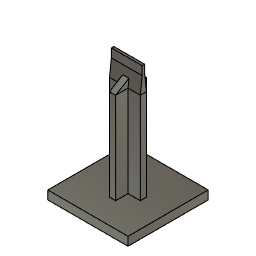
Base apoio braço (Autodesk Fusion 360 design; units mm, degrees)
Autodesk Fusion 360 part; units mm, degrees
sketch "Sketch1" plane through (0, 0, 0) normal (0, 0, 1) x (1, 0, 0)
  line L0 (0, 0) -> (65, 0)
  line L1 (65, 0) -> (65, 65)
  line L2 (65, 65) -> (0, 65)
  line L3 (0, 65) -> (0, 0)
  line L4 (20, 30) -> (45, 30)
  line L5 (45, 30) -> (45, 35)
  line L6 (45, 35) -> (20, 35)
  line L7 (20, 35) -> (20, 30)
  line L8 (30, 20) -> (35, 20)
  line L9 (35, 20) -> (35, 45)
  line L10 (35, 45) -> (30, 45)
  line L11 (30, 45) -> (30, 20)
  dimension "d1" = 65
  dimension "d2" = 65
  dimension "d3" = 25
  dimension "d4" = 5
  dimension "d5" = 5
  dimension "d6" = 25
  constraint horizontal L0
  constraint vertical L1
  constraint horizontal L2
  constraint vertical L3
  constraint coincident L0.start L3.end
  constraint horizontal L4
  constraint vertical L5
  constraint horizontal L6
  constraint vertical L7
  constraint horizontal L8
  constraint vertical L9
  constraint horizontal L10
  constraint vertical L11
  measures "d1" distance of L0.start L0.end
  measures "d2" distance of L0.start L2.end
  measures "d3" distance of L4.start L4.end
  measures "d4" distance of L4.start L6.end
  measures "d5" distance of L8.start L8.end
  measures "d6" distance of L8.start L10.end
extrude "Extrude1" add sketch "Sketch1" against normal blind 7 makes body 1
sketch "Sketch2" plane through (0, 0, 0) normal (0, 0, 1) x (-1, 0, 0)
  line L0 (-30, -35) -> (-30, -45)
  line L1 (-30, -45) -> (-35, -45)
  line L2 (-35, -45) -> (-35, -35)
  line L3 (-35, -35) -> (-45, -35)
  line L4 (-45, -35) -> (-45, -30)
  line L5 (-45, -30) -> (-35, -30)
  line L6 (-35, -30) -> (-35, -20)
  line L7 (-35, -20) -> (-30, -20)
  line L8 (-30, -20) -> (-30, -30)
  line L9 (-30, -30) -> (-20, -30)
  line L10 (-20, -30) -> (-20, -35)
  line L11 (-20, -35) -> (-30, -35)
  line L12 (0, -65) -> (0, 0)
  line L13 (0, 0) -> (-65, 0)
  line L14 (-65, 0) -> (-65, -65)
  line L15 (-65, -65) -> (0, -65)
extrude "Extrude2" add sketch "Sketch2" along normal blind 80 separate body contours L0 L1 L2 L3 L4 L5 L6 L7 L8 L9 L10 L11 makes body 2
sketch "Sketch3" plane through (0, 0, 0) normal (1, 0, 0) x (0, 1, 0)
  line L0 (0, 90) -> (1.5, 103)
  line L1 (0, 90) -> (12.9047, 90) construction
  line L2 (0, 90) -> (5, 90)
  line L3 (5, 90) -> (3.5, 103)
  line L4 (5, 90) -> (18.0144, 90) construction
  line L5 (1.5, 103) -> (1.5, 110)
  line L6 (1.5, 110) -> (3.5, 110)
  line L7 (3.5, 110) -> (3.5, 103)
  dimension "d11" = 83.418
  dimension "d14" = 7
  dimension "d15" = 2
  constraint horizontal L1
  constraint coincident L1 L2.end
  constraint horizontal L4
  constraint vertical L5
  constraint perpendicular L5 L6
  measures "d11" angle of L0 L1
  measures "d14" distance of L0.end L5.end
  measures "d15" distance of L5.end L6.end
extrude "Extrude3" add sketch "Sketch3" along normal blind 25 separate body makes body 3
move_body "Move1" bodies 3 to x (1, 0, 0) y (0, 1, 0) z (0, 0, 1) at (20, 30, -10)
sketch "Sketch4" plane through (0, 0, 0) normal (1, 0, 0) x (0, 1, 0)
  line L0 (20, 86.5) -> (20, 80)
  line L1 (20, 80) -> (30.7531, 86.5)
  line L2 (34.2712, 86.5) -> (45, 80)
  line L3 (34.2712, 86.5) -> (35, 80)
  line L4 (35, 80) -> (45, 80)
  line L5 (30.7531, 86.5) -> (30, 80)
  line L6 (30, 80) -> (20, 80)
  constraint perpendicular L0 L6
extrude "Extrude4" add sketch "Sketch4" along normal blind 5 separate body makes body 4 at (3.3333, 23.5844, 82.1667) makes body 5 at (1.6667, 37.8475, 84.3333)
move_body "Move2" bodies 4 5 to x (1, 0, 0) y (0, 1, 0) z (0, 0, 1) at (30, 0, 0)
sketch "Sketch5" plane through (0, 0, 0) normal (1, 0, 0) x (0, 1, 0)
move_body "Move3" bodies 5 4 3 to x (1, 0, 0) y (0, 1, 0) z (0, 0, 1) at (0, 30, 0)
extrude "Extrude5" cut 1 faces at (41.6667, 31.6667, 80) along direction (0, 0, -1) blind 6 on bodies 2 bodies 2
move_body "Move4" bodies 3 5 4 to x (1, 0, 0) y (0, 1, 0) z (0, 0, 1) at (0, -30, -6)
